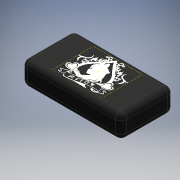
# Autodesk Inventor part: LiPo
Saved by Autodesk Inventor 2016 (Build 200138000, 138)
## iProperties
Created: 2016-09-30
Part Number: LiPo
Material: 一般
Document SubType Name: Modeling
Designer: KOTA-NPC2
Density: 1 g/cm^3
Appearance: 既定
Author: KOTA-NPC2
Autodesk Inventor part; units mm, degrees
ref_plane "YZ Plane" through (0, 0, 0) normal (1, 0, 0) x (0, 1, 0)
ref_plane "XZ Plane" through (0, 0, 0) normal (0, 1, 0) x (-1, 0, 0)
ref_plane "XY Plane" through (0, 0, 0) normal (0, 0, 1) x (1, 0, 0)
sketch "スケッチ2" plane through (0, 0, 0) normal (0, 0, 1) x (1, 0, 0)
  line L0 (-17, 9) -> (17, 9)
  line L1 (17, 9) -> (17, -9)
  line L2 (17, -9) -> (-17, -9)
  line L3 (-17, -9) -> (-17, 9)
  line L4 (-17, 9) -> (17, -9) construction
  line L5 (17, 9) -> (-17, -9) construction
  point P0 (0, 0)
  dimension "d0" = 34
  dimension "d1" = 18
  constraints: 12 end point, 2 midpoint, 2 parallel, 1 horizontal, 1 perpendicular
  measures "d0" distance of L1.end L2.end
  measures "d1" distance of L2.end L0.start
extrude "押し出し1" add sketch "スケッチ2" along normal blind 8
fillet "フィレット1" radius 2 12 edges at (0, -9, 0) (-17, 0, 0) (0, 9, 0) (17, 0, 0) (17, 0, 8) (17, -9, 4) (17, 9, 4) (0, 9, 8) (0, -9, 8) (-17, 0, 8) (-17, -9, 4) (-17, 9, 4)
sketch "スケッチ3" plane through (0, 0, 8) normal (0, 0, 1) x (1, 0, 0)
  line L0 (-8.3616, 6.929) -> (8.3481, 6.929) construction
  line L1 (8.3481, 6.929) -> (8.3481, -6.9758) construction
  line L2 (8.3481, -6.9758) -> (-8.3616, -6.9758) construction
  line L3 (-8.3616, -6.9758) -> (-8.3616, 6.929) construction
  point P0 (0, 0)
  constraints: 2 other
sketch "スケッチ4" plane through (0, 0, 0) normal (0, 0, -1) x (-1, 0, 0)
  line L0 (-8.5496, 7.0043) -> (8.4479, 7.0043) construction
  line L1 (8.4479, 7.0043) -> (8.4479, -7.14) construction
  line L2 (8.4479, -7.14) -> (-8.5496, -7.14) construction
  line L3 (-8.5496, -7.14) -> (-8.5496, 7.0043) construction
  point P0 (0, 0)
  constraints: 2 other
